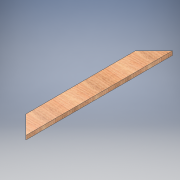
# Autodesk Inventor part: Side Border
Saved by Autodesk Inventor 2017 (Build 210142000, 142)
## iProperties
Created: 2019-02-16
Part Number: Side Border
Material: Generic
Document SubType Name: Modeling
Designer: Mitch
Density: 1 g/cm^3
Appearance: Birch - Natural Polished
Author: Mitch
Autodesk Inventor part; units mm, degrees
ref_plane "YZ Plane" through (0, 0, 0) normal (1, 0, 0) x (0, 1, 0)
ref_plane "XZ Plane" through (0, 0, 0) normal (0, 1, 0) x (-1, 0, 0)
ref_plane "XY Plane" through (0, 0, 0) normal (0, 0, 1) x (1, 0, 0)
sketch "Sketch1" plane through (0, 0, 0) normal (0, 1, 0) x (-1, 0, 0)
  line L0 (88.9, -88.9) -> (88.9, -614.3625)
  line L1 (0, -703.2625) -> (0, 0)
  line L2 (0, 0) -> (88.9, -88.9)
  line L3 (0, -703.2625) -> (88.9, -614.3625)
  dimension "d4" = 703.2625
  dimension "d5" = 45
  dimension "d6" = 45
  dimension "d7" = 88.9
  constraints: 8 end point, 1 parallel
  measures "d4" distance of L1.start L1.end
  measures "d5" angle of L2 L1
  measures "d6" angle of L3 L1
  measures "d7" horizontal distance of L1.start L0.end
extrude "Extrusion1" add sketch "Sketch1" along normal blind 19.05
body "Solid1"
